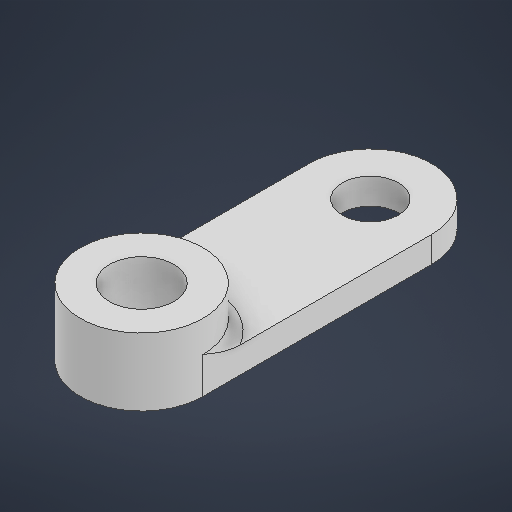
# Autodesk Inventor part: BackSen-TPUPart
Saved by Autodesk Inventor 2027 (Build 310192000, 192)
## iProperties
Created: 2026-06-06
Part Number: BackSen-TPUPart
Material: Všeobecné
Document SubType Name: Modeling
Designer: Vadim
Density: 1 g/cm^3
Appearance: Výchozí
Author: Vadim
Autodesk Inventor part; units mm, degrees
ref_plane "YZ Plane" through (0, 0, 0) normal (1, 0, 0) x (0, 1, 0)
ref_plane "XZ Plane" through (0, 0, 0) normal (0, 1, 0) x (-1, 0, 0)
ref_plane "XY Plane" through (0, 0, 0) normal (0, 0, 1) x (1, 0, 0)
sketch "Náčrt1" plane through (0, 0, 0) normal (0, 1, 0) x (-1, 0, 0)
  circle A0 centre (0, 0) radius 2.95
  circle A1 centre (0, 11) radius 2.95
  circle A2 centre (0, 0) radius 1.35
  circle A3 centre (0, 11) radius 1.55
  line L0 (2.95, 11) -> (2.95, 0)
  line L1 (-2.95, 0) -> (-2.95, 11)
  dimension "d0" = 5.9
  dimension "d1" = 5.9
  dimension "d2" = 11
  dimension "d3" = 2.7
  dimension "d4" = 3.1
  constraints: 4 centre point, 4 end point, 4 point on circle, 4 tangent, 3 coincident, 1 vertical alignment
  measures "d0" diameter of A1
  measures "d1" diameter of A0
  measures "d2" distance of point (0, 0) A1.centre
  measures "d3" diameter of A2
  measures "d4" diameter of A3
extrude "Vysunutí1" add sketch "Náčrt1" along normal blind 1.25 contours A0 | A0 L1 A1 L0
extrude "Vysunutí2" add sketch "Náčrt1" along normal blind 3.25 contours A1
chamfer "Zkosení1" distance 0.5 angle 45 1 edges at (1.55, 0, 11)
fillet "Zaoblení1" radius 0.5 1 edges at (0, 1.25, 8.05)
equation "\"d1\" = d0"
